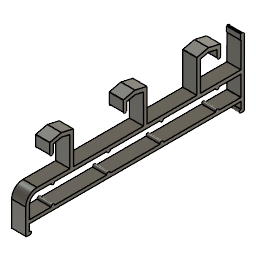
RielTriple (Autodesk Fusion 360 design; units mm, degrees)
part number: 2025-12-27-18-23-46-747
Autodesk Fusion 360 part; units mm, degrees
sketch "Boceto1" plane through (0, 0, 0) normal (1, 0, 0) x (0, 1, 0)
  line L0 (2.5, -7.3) -> (2.5, -2.6)
  line L1 (2.5, -2.6) -> (152.3, -2.5)
  line L2 (152.3, -2.5) -> (152.3032, -7.3069)
  line L3 (154.6552, -8.9997) -> (154.624, 37.7495)
  line L4 (153.173, 39.1986) -> (152.3023, 39.198)
  line L5 (152.2824, 34.8564) -> (152.2, 16.9)
  line L6 (152.2, 16.9) -> (123.5219, 16.8809)
  line L7 (123.5219, 16.8809) -> (123.5081, 37.6781)
  line L8 (123.5852, 37.7756) -> (129.2904, 39.1126)
  line L9 (129.2904, 39.1126) -> (135.2262, 37.7662)
  line L10 (135.3041, 37.6687) -> (135.3075, 32.5991)
  line L11 (137.8925, 32.6009) -> (137.8868, 39.901)
  line L12 (137.8089, 39.9985) -> (129.2904, 41.9307)
  line L13 (129.2904, 41.9307) -> (121.0848, 40.0077)
  line L14 (121.0076, 39.9102) -> (121.023, 16.8809)
  line L15 (121.023, 16.8809) -> (85.8383, 16.8574)
  line L16 (85.8383, 16.8574) -> (85.8229, 39.9098)
  line L17 (85.7451, 40.0072) -> (77.2651, 41.9307)
  line L18 (77.2651, 41.9307) -> (69.0595, 40.0077)
  line L19 (68.9823, 39.9102) -> (68.9873, 32.5002)
  line L20 (71.5218, 32.4984) -> (71.5253, 37.6782)
  line L21 (71.6025, 37.7755) -> (77.3077, 39.1126)
  line L22 (77.3077, 39.1126) -> (83.2041, 37.7751)
  line L23 (83.282, 37.6777) -> (83.2959, 16.8574)
  line L24 (83.2959, 16.8574) -> (33.815, 16.8243)
  line L25 (33.815, 16.8243) -> (33.7996, 39.9098)
  line L26 (33.7217, 40.0072) -> (25.2418, 41.9307)
  line L27 (25.2418, 41.9307) -> (17.0361, 40.0076)
  line L28 (16.9589, 39.9104) -> (16.9539, 32.5002)
  line L29 (19.4954, 32.5002) -> (19.4954, 37.6782)
  line L30 (19.5726, 37.7756) -> (25.2418, 39.1042)
  line L31 (25.2418, 39.1042) -> (31.101, 37.7751)
  line L32 (31.1789, 37.6776) -> (31.1789, 16.85)
  line L33 (31.1789, 16.85) -> (8.0385, 16.9613)
  line L34 (0, 8.9614) -> (0, -9)
  arc A0 (16.9539, 32.5019) -> (19.4954, 32.5002) centre (18.2246, 32.5002) ccw
  arc A1 (68.9873, 32.5002) -> (71.5218, 32.4984) centre (70.2545, 32.4993) ccw
  arc A2 (135.3075, 32.5991) -> (137.8925, 32.6009) centre (136.6, 32.6) ccw
  arc A3 (8.0385, 16.9613) -> (0, 8.9614) centre (8, 8.9614) ccw
  arc A4 (8.0259, 14.3527) -> (2.6087, 8.9614) centre (8, 8.9614) ccw
  line L35 (31.1599, 14.2414) -> (33.8032, 14.2156)
  line L36 (83.2968, 14.2487) -> (85.8392, 14.2487)
  line L37 (121.0238, 14.2722) -> (123.5228, 14.2722)
  line L38 (152.2018, 14.1913) -> (152.2112, 0.101)
  line L39 (2.6087, 0.0012) -> (2.6087, 8.9614)
  arc A5 (2.6087, 0.0012) -> (2.7087, -0.0988) centre (2.7087, 0.0012) ccw
  arc A6 (152.2018, 14.1913) -> (152.1017, 14.2913) centre (152.1018, 14.1913) ccw
  arc A7 (152.1113, 0.0009) -> (152.2112, 0.101) centre (152.1112, 0.1009) ccw
  arc A8 (17.0361, 40.0076) -> (16.9589, 39.9104) centre (17.0589, 39.9103) ccw
  arc A9 (33.7996, 39.9098) -> (33.7217, 40.0072) centre (33.6996, 39.9097) ccw
  arc A10 (31.1789, 37.6776) -> (31.101, 37.7751) centre (31.0789, 37.6776) ccw
  arc A11 (19.5726, 37.7756) -> (19.4954, 37.6782) centre (19.5954, 37.6782) ccw
  arc A12 (71.6025, 37.7755) -> (71.5253, 37.6782) centre (71.6253, 37.6782) ccw
  arc A13 (69.0595, 40.0077) -> (68.9823, 39.9102) centre (69.0823, 39.9103) ccw
  arc A14 (85.8229, 39.9098) -> (85.7451, 40.0072) centre (85.7229, 39.9097) ccw
  arc A15 (83.282, 37.6777) -> (83.2041, 37.7751) centre (83.182, 37.6776) ccw
  arc A16 (137.8868, 39.901) -> (137.8089, 39.9985) centre (137.7868, 39.9009) ccw
  arc A17 (135.3041, 37.6687) -> (135.2262, 37.7662) centre (135.2041, 37.6686) ccw
  arc A18 (121.0848, 40.0077) -> (121.0076, 39.9102) centre (121.1076, 39.9103) ccw
  arc A19 (123.5852, 37.7756) -> (123.5081, 37.6781) centre (123.6081, 37.6782) ccw
  line L40 (2.5, -7.3) -> (3, -7.3)
  line L41 (0.5, -9.5) -> (3, -9.5)
  arc A20 (3, -9.5) -> (3, -7.3) centre (3, -8.4) ccw
  arc A21 (0, -9) -> (0.5, -9.5) centre (0.5, -9) ccw
  line L42 (152.0019, -9.4515) -> (154.2055, -9.45)
  line L43 (152.0005, -7.3071) -> (152.3032, -7.3069)
  arc A22 (152.0005, -7.3071) -> (152.0019, -9.4515) centre (152.0012, -8.3793) ccw
  arc A23 (154.2055, -9.45) -> (154.6552, -8.9997) centre (154.2052, -9) ccw
  line L44 (152.3023, 39.198) -> (152.0998, 39.1989)
  line L45 (151.8989, 38.9998) -> (151.8815, 35.2082)
  line L46 (152.0557, 35.0324) -> (152.1082, 35.0322)
  arc A24 (152.0998, 39.1989) -> (151.8989, 38.9998) centre (152.0989, 38.9989) ccw
  arc A25 (154.624, 37.7495) -> (153.173, 39.1986) centre (153.174, 37.7486) ccw
  arc A26 (152.2824, 34.8564) -> (152.1082, 35.0322) centre (152.1074, 34.8572) ccw
  arc A27 (151.8815, 35.2082) -> (152.0557, 35.0324) centre (152.0565, 35.2074) ccw
  arc A28 (17.8722, 14.3053) -> (20.4921, 14.2972) centre (19.1822, 14.3088) ccw
  arc A29 (94.8722, 14.3053) -> (97.4921, 14.2972) centre (96.1822, 14.3088) ccw
  arc A30 (134.2722, 14.3053) -> (136.8921, 14.2972) centre (135.5822, 14.3088) ccw
  arc A31 (57.2722, 14.3053) -> (59.8921, 14.2972) centre (58.5822, 14.3088) ccw
  line L47 (31.1599, 14.2414) -> (20.4921, 14.2927)
  line L48 (17.8722, 14.3053) -> (8.0259, 14.3527)
  line L49 (83.2968, 14.2487) -> (59.89, 14.2331)
  line L50 (57.2745, 14.2313) -> (33.8032, 14.2156)
  line L51 (121.0238, 14.2722) -> (97.4911, 14.2565)
  line L52 (94.8734, 14.2547) -> (85.8392, 14.2487)
  line L53 (152.1017, 14.2913) -> (136.8919, 14.2811)
  line L54 (134.2726, 14.2793) -> (123.5228, 14.2722)
  arc A32 (20.4928, -0.087) -> (17.9364, -0.0887) centre (19.2145, -0.0291) ccw
  arc A33 (59.8558, -0.0607) -> (57.197, -0.0625) centre (58.5264, -0.0037) ccw
  arc A34 (97.4772, -0.0356) -> (94.9603, -0.0373) centre (96.2187, 0.0563) ccw
  arc A35 (136.7444, -0.0094) -> (134.2956, -0.011) centre (135.52, 0.07) ccw
  line L55 (152.1113, 0.0009) -> (136.7444, -0.0094)
  line L56 (134.2956, -0.011) -> (97.4772, -0.0356)
  line L57 (94.9603, -0.0373) -> (59.8558, -0.0607)
  line L58 (57.197, -0.0625) -> (20.4928, -0.087)
  line L59 (17.9364, -0.0887) -> (2.7087, -0.0988)
  dimension "d1" = 8
  dimension "d3" = 0.1
  dimension "d4" = 0.1
  dimension "d5" = 0.1
  dimension "d6" = 0.5
  dimension "d7" = 0.45
  dimension "d8" = 0.2
  dimension "d9" = 1.45
  dimension "d10" = 0.175
  dimension "d13" = 77
  dimension "d14" = 0
  dimension "d17" = 39.4
  dimension "d18" = 0
  dimension "d21" = -37.6
  dimension "d22" = 0
  constraint perpendicular L1 L2
  constraint perpendicular L1 L3
  constraint perpendicular L3 L4
  constraint perpendicular L3 L6
  constraint perpendicular L6 L7
  constraint parallel L7 L10
  constraint parallel L9 L12
  constraint parallel L8 L13
  constraint perpendicular L6 L14
  constraint perpendicular L14 L15
  constraint perpendicular L15 L16
  constraint parallel L12 L17
  constraint parallel L13 L18
  constraint parallel L16 L19
  constraint parallel L18 L21
  constraint parallel L17 L22
  constraint perpendicular L15 L23
  constraint perpendicular L14 L24
  constraint perpendicular L24 L25
  constraint parallel L17 L26
  constraint parallel L18 L27
  constraint parallel L27 L30
  constraint parallel L26 L31
  constraint parallel L29 L32
  constraint coincident L28.end A0
  constraint coincident L28 A0.start
  constraint tangent L33 A3
  constraint tangent L34 A3
  constraint perpendicular L1 L38
  constraint perpendicular L3 L55
  constraint tangent A4 L39
  constraint tangent A5 L55
  constraint tangent L39 A5
  constraint concentric A3 A4
  constraint tangent A4 L47
  constraint tangent A6 L53
  constraint tangent L38 A6
  constraint tangent L38 A7
  constraint tangent A7 L55
  constraint equal A6 A7
  constraint tangent L27 A8
  constraint tangent L28 A8
  constraint tangent L25 A9
  constraint tangent L26 A9
  constraint equal A8 A9
  constraint tangent L31 A10
  constraint tangent L32 A10
  constraint equal A8 A10
  constraint tangent L29 A11
  constraint tangent L30 A11
  constraint equal A8 A11
  constraint tangent L20 A12
  constraint tangent L21 A12
  constraint equal A8 A12
  constraint tangent L18 A13
  constraint tangent L19 A13
  constraint equal A8 A13
  constraint tangent L16 A14
  constraint tangent L17 A14
  constraint equal A8 A14
  constraint tangent L22 A15
  constraint tangent L23 A15
  constraint equal A8 A15
  constraint tangent L11 A16
  constraint tangent L12 A16
  constraint equal A8 A16
  constraint tangent L9 A17
  constraint tangent L10 A17
  constraint equal A8 A17
  constraint tangent L13 A18
  constraint tangent L14 A18
  constraint equal A8 A18
  constraint tangent L7 A19
  constraint tangent L8 A19
  constraint equal A8 A19
  constraint tangent L34 A21
  constraint tangent L41 A21
  constraint perpendicular L3 L42
  constraint perpendicular L2 L43
  constraint tangent L3 A23
  constraint tangent L42 A23
  constraint perpendicular L5 L44
  constraint perpendicular L44 L45
  constraint perpendicular L5 L46
  constraint tangent L44 A24
  constraint tangent L45 A24
  constraint tangent L3 A25
  constraint tangent L4 A25
  constraint tangent L5 A26
  constraint tangent L46 A26
  constraint tangent L45 A27
  constraint tangent L46 A27
  constraint equal A26 A27
  constraint coincident A28.start L47
  constraint coincident A28 L47.end
  constraint collinear L47 L48
  constraint coincident A31 L49.end
  constraint coincident A31 L50.start
  constraint collinear L49 L50
  constraint coincident A29 L51.end
  constraint coincident A29 L52.start
  constraint collinear L51 L52
  constraint coincident A30 L53.end
  constraint coincident A30 L54.start
  constraint collinear L53 L54
  constraint coincident A32.start L55
  constraint coincident A32.end L55
  constraint coincident A33.start L55
  constraint coincident A33.end L55
  constraint coincident A34.start L55
  constraint coincident A34.end L55
  constraint coincident A35.end L55
  constraint collinear L55 L56
  constraint collinear L56 L57
  constraint collinear L57 L58
  constraint collinear L58 L59
  measures "d1" radius of A3
  measures "d3" radius of A5
  measures "d4" radius of A6
  measures "d5" radius of A8
  measures "d6" radius of A21
  measures "d7" radius of A23
  measures "d8" radius of A24
  measures "d9" radius of A25
  measures "d10" radius of A26
extrude "Extruir1" add sketch "Boceto1" along normal blind 10
equation "L = 10 mm"
equation "d25 = L"
